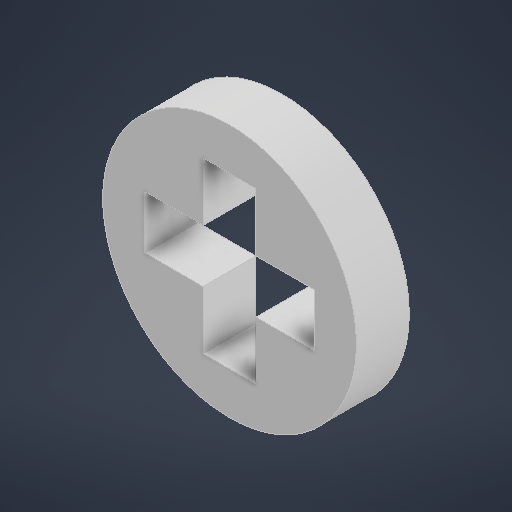
# Autodesk Inventor part: pitahaya6
Saved by Autodesk Inventor 2026.3 (Build 303398000, 398)
## iProperties
Created: 2024-05-08
Part Number: pitahaya6
Material: Generic
Document SubType Name: Modeling
Designer: Wilhelm
Density: 1 g/cm^3
Appearance: Default
Author: Wilhelm
Autodesk Inventor part; units mm, degrees
ref_plane "YZ Plane" through (0, 0, 0) normal (1, 0, 0) x (0, 1, 0)
ref_plane "XZ Plane" through (0, 0, 0) normal (0, 1, 0) x (-1, 0, 0)
ref_plane "XY Plane" through (0, 0, 0) normal (0, 0, 1) x (1, 0, 0)
sketch "Sketch1" plane through (0, 0, 0) normal (0, 0, 1) x (1, 0, 0)
  circle A0 centre (0, 0) radius 6
  circle A1 centre (0, 0) radius 4.1908 construction
  line L0 (-1.25, 4) -> (1.25, 4)
  line L1 (1.25, -4) -> (-1.25, -4)
  line L2 (4, 1.25) -> (4, -1.25)
  line L3 (-4, -1.25) -> (-4, 1.25)
  line L4 (0, 2.7092) -> (0, -2.7092) construction
  line L5 (-2.0091, 0) -> (2.0091, 0) construction
  line L6 (-4, 1.25) -> (-1.25, 1.25)
  line L7 (1.25, 1.25) -> (4, 1.25)
  line L8 (4, -1.25) -> (1.25, -1.25)
  line L9 (-1.25, -1.25) -> (-4, -1.25)
  line L10 (-1.25, -4) -> (-1.25, -1.25)
  line L11 (-1.25, 1.25) -> (-1.25, 4)
  line L12 (1.25, 4) -> (1.25, 1.25)
  line L13 (1.25, -1.25) -> (1.25, -4)
  dimension "d1" = 8
  dimension "d2" = 8
  dimension "d3" = 2.5
  dimension "d4" = 2.5
  dimension "d7" = 12
  constraints: 28 end point, 10 parallel, 6 perpendicular, 3 coincident, 3 horizontal, 2 horizontal alignment, 2 midpoint, 2 vertical alignment, 1 centre point, 1 vertical, 7 other
  measures "d1" distance between parallel lines of L2 L3
  measures "d2" distance between parallel lines of L1 L0
  measures "d3" distance of L3.start L3.end
  measures "d4" distance of L0.start L0.end
  measures "d7" diameter of A0
extrude "Extrusion1" add sketch "Sketch1" along normal mid plane 2.5
body "Solid1"
